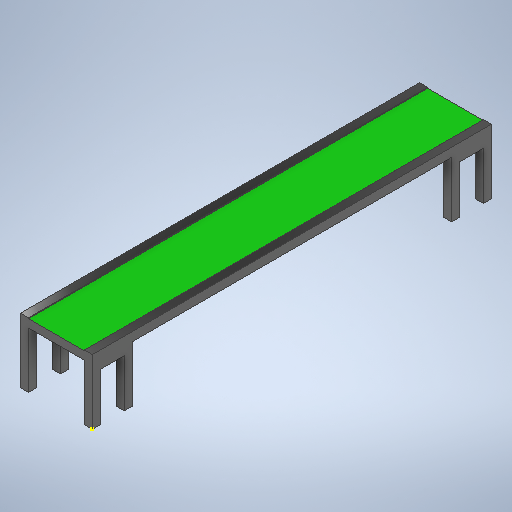
# Autodesk Inventor part: B_Transportadora_Recta_5m
Saved by Autodesk Inventor 2025.2 (Build 292293000, 293)
## iProperties
Created: 2025-01-23
Part Number: B_Transportadora_Recta_5m
Material: Aluminum 6061
Document SubType Name: Modeling
Designer: Proyectos
Density: 2.7 g/cm^3
Appearance: Engine Turned
Author: Proyectos
Autodesk Inventor part; units mm, degrees
ref_plane "YZ Plane" through (0, 0, 0) normal (1, 0, 0) x (0, 1, 0)
ref_plane "XZ Plane" through (0, 0, 0) normal (0, 1, 0) x (-1, 0, 0)
ref_plane "XY Plane" through (0, 0, 0) normal (0, 0, 1) x (1, 0, 0)
sketch "Sketch9" plane through (0, 0, 0) normal (0, 1, 0) x (-1, 0, 0)
  line L0 (0, 0) -> (900, 0)
  line L1 (900, 0) -> (900, -5000)
  line L2 (900, -5000) -> (0, -5000)
  line L3 (0, -5000) -> (0, 0)
  line L4 (900, -5000) -> (800, -5000)
  line L5 (800, -5000) -> (800, 0)
  line L6 (800, 0) -> (900, 0)
  line L7 (900, 0) -> (900, -5000)
  line L8 (0, -5000) -> (100, -5000)
  line L9 (100, -5000) -> (100, 0)
  line L10 (100, 0) -> (0, 0)
  line L11 (0, 0) -> (0, -5000)
  dimension "d70" = 900
  dimension "d71" = 100
  dimension "d72" = 100
  constraints: 24 end point, 6 parallel, 3 horizontal, 3 perpendicular
  measures "d70" distance of L1.end L2.end
  measures "d71" distance of L5.end L6.end
  measures "d72" distance of L10.end L9.end
extrude "Extrusion6" add sketch "Sketch9" along normal blind 1100 contours L0 L9 L2 L3 | L0 L1 L2 L5
sketch "Sketch10" plane through (0, 0, 0) normal (1, 0, 0) x (0, 0, -1)
  line L0 (0, 0) -> (0, 1100) projected
  line L1 (0, 1100) -> (5000, 1100)
  line L2 (5000, 1100) -> (5000, 600)
  line L3 (5000, 600) -> (0, 600)
  line L4 (0, 600) -> (0, 1100)
  line L5 (0, 1100) -> (5000, 1100)
  line L6 (5000, 1100) -> (5000, 700)
  line L7 (5000, 700) -> (0, 700)
  line L8 (0, 700) -> (0, 1100)
  line L9 (0, 1100) -> (5000, 1100)
  line L10 (5000, 1100) -> (5000, 800)
  line L11 (5000, 800) -> (0, 800)
  line L12 (0, 800) -> (0, 1100)
  line L13 (5000, 0) -> (0, 0) projected
  line L14 (0, 0) -> (500, 0)
  line L15 (500, 0) -> (500, 600)
  line L16 (500, 600) -> (0, 600)
  line L17 (0, 600) -> (0, 0)
  line L18 (5000, 0) -> (4500, 0)
  line L19 (4500, 0) -> (4500, 600)
  line L20 (4500, 600) -> (5000, 600)
  line L21 (5000, 600) -> (5000, 0)
  point P0 (0, 800)
  dimension "d83" = 500
  dimension "d84" = 500
  dimension "d85" = 600
  dimension "d86" = 600
  constraints: 40 end point, 10 parallel, 5 horizontal, 5 perpendicular
  measures "d83" distance of L15.end L16.end
  measures "d84" distance of L19.end L20.end
  measures "d85" distance of L14.end L15.end
  measures "d86" distance of L18.end L19.end
extrude "Extrusion7" add sketch "Sketch10" against normal blind 900 contours L0 L11 L2 L7
sketch "Sketch11" plane through (0, 0, 0) normal (1, 0, 0) x (0, 0, -1)
  point P0 (0, 0)
sketch "Sketch12" plane through (0, 0, 0) normal (1, 0, 0) x (0, 0, -1)
  line L0 (0, 0) -> (500, 0)
  line L1 (500, 0) -> (500, 600)
  line L2 (500, 600) -> (0, 600)
  line L3 (0, 600) -> (0, 0)
  line L4 (0, 0) -> (5000, 0) projected
  line L5 (5000, 0) -> (4500, 0)
  line L6 (4500, 0) -> (4500, 600)
  line L7 (4500, 600) -> (5000, 600)
  line L8 (5000, 600) -> (5000, 0)
  line L9 (500, 600) -> (4500, 600)
  dimension "d89" = 500
  dimension "d91" = 600
  dimension "d92" = 500
  dimension "d93" = 600
  constraints: 18 end point, 4 parallel, 2 horizontal, 2 perpendicular
  measures "d89" distance of L1.end L2.end
  measures "d91" distance of L0.end L1.end
  measures "d92" distance of L6.end L7.end
  measures "d93" distance of L5.end L6.end
extrude "Extrusion8" cut sketch "Sketch12" against normal blind 900 contours L1 L9 L6 L4
sketch "Sketch13" plane through (0, 1100, 0) normal (0, 1, 0) x (1, 0, 0)
  line L0 (-900, 5000) -> (-900, 0) projected
  line L1 (0, 4500) -> (0, 5000) projected
  line L2 (-900, 0) -> (0, 0)
  line L3 (0, 0) -> (0, 5000)
  line L4 (0, 5000) -> (-900, 5000)
  line L5 (-900, 5000) -> (-900, 0)
  constraints: 8 end point, 2 parallel, 1 horizontal, 1 perpendicular
extrude "Extrusion9" cut sketch "Sketch13" against normal blind 290
sketch "Sketch14" plane through (0, 0, 0) normal (1, 0, 0) x (0, 0, -1)
  line L0 (5000, 810) -> (0, 810) projected
  line L1 (0, 0) -> (0, 810) projected
  line L2 (0, 0) -> (500, 0) projected
  line L3 (500, 0) -> (500, 600) projected
  line L4 (500, 600) -> (4500, 600) projected
  line L5 (4500, 600) -> (4500, 0) projected
  line L6 (4500, 0) -> (5000, 0) projected
  line L7 (5000, 0) -> (5000, 810) projected
  line L8 (0, 0) -> (100, 0)
  line L9 (100, 0) -> (500, 0)
  line L10 (500, 0) -> (0, 0) projected
  line L11 (500, 0) -> (400, 0)
  line L12 (100, 0) -> (400, 0)
  line L13 (400, 0) -> (400, 600)
  line L14 (400, 600) -> (100, 600)
  line L15 (100, 600) -> (100, 0)
  line L16 (4500, 0) -> (4600, 0)
  line L17 (5000, 0) -> (4900, 0)
  line L18 (5000, 0) -> (4500, 0) projected
  line L19 (4600, 0) -> (4900, 0)
  line L20 (4900, 0) -> (4900, 600)
  line L21 (4900, 600) -> (4600, 600)
  line L22 (4600, 600) -> (4600, 0)
  line L23 (0, 700) -> (5000, 700) projected
  line L24 (500, 600) -> (4500, 600)
  line L25 (4500, 600) -> (4500, 700)
  line L26 (4500, 700) -> (500, 700)
  line L27 (500, 700) -> (500, 600)
  point P0 (500, 700)
  dimension "d98" = 100
  dimension "d99" = 100
  dimension "d100" = 100
  dimension "d101" = 100
  constraints: 34 end point, 6 parallel, 5 point on line, 3 horizontal, 3 perpendicular, 1 collinear
  measures "d98" distance of L1.start L8.end
  measures "d99" distance of L2.end L11.end
  measures "d100" distance of L5.end L16.end
  measures "d101" distance of L6.end L17.end
extrude "Extrusion10" cut sketch "Sketch14" against normal through all contours L25 L4 L27 L23 | L6 L22 L21 L20 | L15 L14 L13 L2
body "Solid2"
